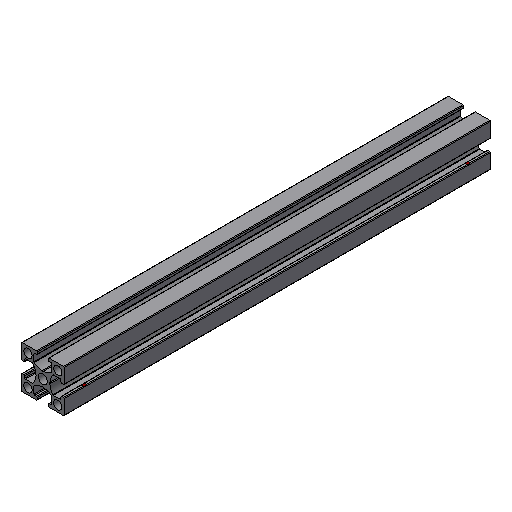
# Autodesk Inventor part: TL20240901-10320CV-101
Saved by Autodesk Inventor 2022.5 (Build 265521000, 521)
## iProperties
Category: FOLLOWER UNIT ASSY
Company: 현대 트랜시스
Created: 2022-11-16
Part Number: TL20240901-10320CV-101
User Status: 2
Material: AL6061
Description: 1
Document SubType Name: Modeling
Designer: domyung.kim
Density: 2.71 g/cm^3
Appearance: 기본값
Project: MEa-PJT 2LINE
Checked By: 김형민
Engr Approved By: 김형민
Mfg Approved By: 호상태
Stock Number: 101
MAKER: DY PROFILE
Detail Description: Purchased processed products
Title: AL PROFILE/DP2020-200L
Author: 최신영
Revision Number: B
Subject: MEa차종 시트조립2라인
Autodesk Inventor part; units mm, degrees
ref_plane "YZ Plane" through (0, 0, 0) normal (1, 0, 0) x (0, 1, 0)
ref_plane "XZ Plane" through (0, 0, 0) normal (0, 1, 0) x (-1, 0, 0)
ref_plane "XY Plane" through (0, 0, 0) normal (0, 0, 1) x (1, 0, 0)
sketch "스케치3" plane through (0, 0, 0) normal (0, 0, 1) x (1, 0, 0)
  line L0 (-11.1989, 0) -> (11.1989, 0)
  circle A0 centre (0, 0) radius 2.15
  line L1 (4.15, 4.9427) -> (4.15, 8.2)
  arc A1 (4.15, 8.2) -> (3.85, 8.5) centre (3.85, 8.2) ccw
  line L2 (3.85, 8.5) -> (2.95, 8.5)
  arc A2 (2.65, 8.8) -> (2.95, 8.5) centre (2.95, 8.8) ccw
  line L3 (2.65, 8.8) -> (2.65, 9.7)
  arc A3 (2.95, 10) -> (2.65, 9.7) centre (2.95, 9.7) ccw
  line L4 (2.95, 10) -> (9.7, 10)
  arc A4 (10, 9.7) -> (9.7, 10) centre (9.7, 9.7) ccw
  line L5 (10, 9.7) -> (10, 2.95)
  arc A5 (9.7, 2.65) -> (10, 2.95) centre (9.7, 2.95) ccw
  line L6 (9.7, 2.65) -> (8.8, 2.65)
  arc A6 (8.5, 2.95) -> (8.8, 2.65) centre (8.8, 2.95) ccw
  line L7 (8.5, 2.95) -> (8.5, 3.85)
  arc A7 (8.5, 3.85) -> (8.2, 4.15) centre (8.2, 3.85) ccw
  line L8 (8.2, 4.15) -> (4.9427, 4.15)
  arc A8 (4.9427, 4.15) -> (4.7078, 4.0366) centre (4.9427, 3.85) ccw
  arc A9 (4.7078, 4.0366) -> (3.3073, 0.3073) centre (9.7908, 0) ccw
  line L9 (3.3073, 0.3073) -> (3, 0)
  line L10 (3, 0) -> (3.3073, -0.3073)
  arc A10 (3.3073, -0.3073) -> (4.7078, -4.0366) centre (9.7908, 0) ccw
  arc A11 (4.7078, -4.0366) -> (4.9427, -4.15) centre (4.9427, -3.85) ccw
  line L11 (4.9427, -4.15) -> (8.2, -4.15)
  arc A12 (8.2, -4.15) -> (8.5, -3.85) centre (8.2, -3.85) ccw
  line L12 (8.5, -3.85) -> (8.5, -2.95)
  arc A13 (8.8, -2.65) -> (8.5, -2.95) centre (8.8, -2.95) ccw
  line L13 (8.8, -2.65) -> (9.7, -2.65)
  arc A14 (10, -2.95) -> (9.7, -2.65) centre (9.7, -2.95) ccw
  line L14 (10, -2.95) -> (10, -9.7)
  arc A15 (9.7, -10) -> (10, -9.7) centre (9.7, -9.7) ccw
  line L15 (9.7, -10) -> (2.95, -10)
  arc A16 (2.65, -9.7) -> (2.95, -10) centre (2.95, -9.7) ccw
  line L16 (2.65, -9.7) -> (2.65, -8.8)
  arc A17 (2.95, -8.5) -> (2.65, -8.8) centre (2.95, -8.8) ccw
  line L17 (2.95, -8.5) -> (3.85, -8.5)
  arc A18 (3.85, -8.5) -> (4.15, -8.2) centre (3.85, -8.2) ccw
  line L18 (4.15, -8.2) -> (4.15, -4.9427)
  arc A19 (4.15, -4.9427) -> (4.0366, -4.7078) centre (3.85, -4.9427) ccw
  arc A20 (4.0366, -4.7078) -> (0.3073, -3.3073) centre (0, -9.7908) ccw
  line L19 (0.3073, -3.3073) -> (0, -3)
  line L20 (0, -3) -> (-0.3073, -3.3073)
  arc A21 (-0.3073, -3.3073) -> (-4.0366, -4.7078) centre (0, -9.7908) ccw
  arc A22 (-4.0366, -4.7078) -> (-4.15, -4.9427) centre (-3.85, -4.9427) ccw
  line L21 (-4.15, -4.9427) -> (-4.15, -8.2)
  arc A23 (-4.15, -8.2) -> (-3.85, -8.5) centre (-3.85, -8.2) ccw
  line L22 (-3.85, -8.5) -> (-2.95, -8.5)
  arc A24 (-2.65, -8.8) -> (-2.95, -8.5) centre (-2.95, -8.8) ccw
  line L23 (-2.65, -8.8) -> (-2.65, -9.7)
  arc A25 (-2.95, -10) -> (-2.65, -9.7) centre (-2.95, -9.7) ccw
  line L24 (-2.95, -10) -> (-9.7, -10)
  arc A26 (-10, -9.7) -> (-9.7, -10) centre (-9.7, -9.7) ccw
  line L25 (-10, -9.7) -> (-10, -2.95)
  arc A27 (-9.7, -2.65) -> (-10, -2.95) centre (-9.7, -2.95) ccw
  line L26 (-9.7, -2.65) -> (-8.8, -2.65)
  arc A28 (-8.5, -2.95) -> (-8.8, -2.65) centre (-8.8, -2.95) ccw
  line L27 (-8.5, -2.95) -> (-8.5, -3.85)
  arc A29 (-8.5, -3.85) -> (-8.2, -4.15) centre (-8.2, -3.85) ccw
  line L28 (-8.2, -4.15) -> (-4.9427, -4.15)
  arc A30 (-4.9427, -4.15) -> (-4.7078, -4.0366) centre (-4.9427, -3.85) ccw
  arc A31 (-4.7078, -4.0366) -> (-3.3073, -0.3073) centre (-9.7908, 0) ccw
  line L29 (-3.3073, -0.3073) -> (-3, 0)
  line L30 (-3, 0) -> (-3.3073, 0.3073)
  arc A32 (-3.3073, 0.3073) -> (-4.7078, 4.0366) centre (-9.7908, 0) ccw
  arc A33 (-4.7078, 4.0366) -> (-4.9427, 4.15) centre (-4.9427, 3.85) ccw
  line L31 (-4.9427, 4.15) -> (-8.2, 4.15)
  arc A34 (-8.2, 4.15) -> (-8.5, 3.85) centre (-8.2, 3.85) ccw
  line L32 (-8.5, 3.85) -> (-8.5, 2.95)
  arc A35 (-8.8, 2.65) -> (-8.5, 2.95) centre (-8.8, 2.95) ccw
  line L33 (-8.8, 2.65) -> (-9.7, 2.65)
  arc A36 (-10, 2.95) -> (-9.7, 2.65) centre (-9.7, 2.95) ccw
  line L34 (-10, 2.95) -> (-10, 9.7)
  arc A37 (-9.7, 10) -> (-10, 9.7) centre (-9.7, 9.7) ccw
  line L35 (-9.7, 10) -> (-2.95, 10)
  arc A38 (-2.65, 9.7) -> (-2.95, 10) centre (-2.95, 9.7) ccw
  line L36 (-2.65, 9.7) -> (-2.65, 8.8)
  arc A39 (-2.95, 8.5) -> (-2.65, 8.8) centre (-2.95, 8.8) ccw
  line L37 (-2.95, 8.5) -> (-3.85, 8.5)
  arc A40 (-3.85, 8.5) -> (-4.15, 8.2) centre (-3.85, 8.2) ccw
  line L38 (-4.15, 8.2) -> (-4.15, 4.9427)
  arc A41 (-4.15, 4.9427) -> (-4.0366, 4.7078) centre (-3.85, 4.9427) ccw
  arc A42 (-4.0366, 4.7078) -> (-0.3073, 3.3073) centre (0, 9.7908) ccw
  line L39 (-0.3073, 3.3073) -> (0, 3)
  line L40 (0, 3) -> (0.3073, 3.3073)
  arc A43 (0.3073, 3.3073) -> (4.0366, 4.7078) centre (0, 9.7908) ccw
  arc A44 (4.0366, 4.7078) -> (4.15, 4.9427) centre (3.85, 4.9427) ccw
  line L41 (-9.5, 7) -> (-4.5, 7)
  line L42 (-7, 9.5) -> (-7, 4.5)
  circle A45 centre (-7, 7) radius 2
  line L43 (-9.5, -7) -> (-4.5, -7)
  line L44 (-7, -9.5) -> (-7, -4.5)
  circle A46 centre (-7, -7) radius 2
  line L45 (9.5, 7) -> (4.5, 7)
  line L46 (7, 9.5) -> (7, 4.5)
  circle A47 centre (7, 7) radius 2
  circle A48 centre (7, -7) radius 2
  line L47 (7, -9.5) -> (7, -4.5)
  line L48 (9.5, -7) -> (4.5, -7)
  constraints: 98 end point, 88 point on circle, 49 centre point, 2 point on line
extrude "돌출1" add sketch "스케치3" along normal mid plane 200 contours A0 L0 L30 A32 A33 L31 A34 L32 A35 L33 A36 L34 A37 L35 A38 L36 A39 L37 A40 L38 A41 A42 L39 L40 A43 A44 L1 A1 L2 A2 L3 A3 L4 A4 L5 A5 L6 A6 L7 A7 L8 A8 A9 L9 | L0 L10 A10 A11 L11 A12 L12 A13 L13 A14 L14 A15 L15 A16 L16 A17 L17 A18 L18 A19 A20 L19 L20 A21 A22 L21 A23 L22 A24 L23 A25 L24 A26 L25 A27 L26 A28 L27 A29 L28 A30 A31 L29 A0
sketch "Sketch4" plane through (10, -9.7, 100) normal (1, 0, 0) x (0, 0, -1)
  line L0 (0, 12.65) -> (0, 19.4) projected
  line L1 (200, 19.7) -> (0, 19.7) projected
  line L2 (200, 19.4) -> (200, 12.65) projected
  point P0 (100, 9.7)
  point P1 (10, 9.7)
  point P2 (190, 9.7)
  dimension "d2" = 10
  dimension "d3" = 10
  dimension "d4" = 10
  constraints: 1 horizontal alignment
  measures "d2" distance from line of point (10, 9.7) L0
  measures "d3" distance from line of point (10, 9.7) L1
  measures "d4" distance from line of point (190, 9.7) L2
hole "Hole1" at (10, 0, 90) at (10, 0, -90) direction (-1, 0, 0) diameter 5.5 end through all clearance for "Socket Head Cap Screw" size "M5" standard "TS Profile"
equation "\"d4\" = d2"
